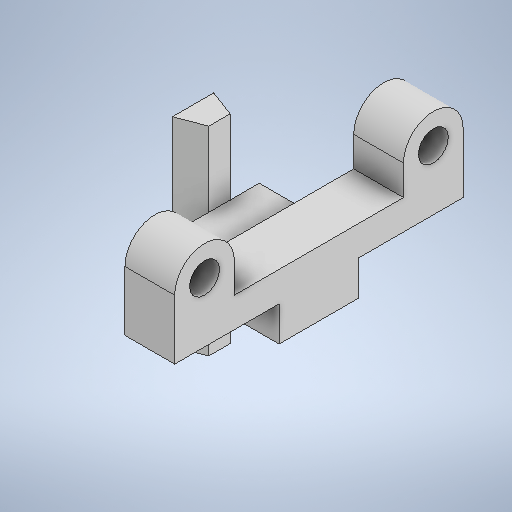
# Autodesk Inventor part: pelvis øvre del
Saved by Autodesk Inventor 2025.1 (Build 291241020, 241B)
## iProperties
Created: 2024-10-22
Part Number: pelvis øvre del
Material: Generic
Document SubType Name: Modeling
Designer: morte
Density: 1 g/cm^3
Appearance: Default
Author: morte
Autodesk Inventor part; units mm, degrees
ref_plane "YZ Plane" through (0, 0, 0) normal (1, 0, 0) x (0, 1, 0)
ref_plane "XZ Plane" through (0, 0, 0) normal (0, 1, 0) x (-1, 0, 0)
ref_plane "XY Plane" through (0, 0, 0) normal (0, 0, 1) x (1, 0, 0)
sketch "Sketch1" plane through (0, 0, 0) normal (1, 0, 0) x (0, 1, 0)
  line L0 (0, 0) -> (0, 8.5)
  line L1 (0, 14.5) -> (6, 14.5)
  line L2 (0, 0) -> (0, -8.5)
  line L3 (0, -14.5) -> (6, -14.5)
  line L4 (6, -14.5) -> (6, -8.5)
  line L5 (6, -8.5) -> (0, -8.5)
  line L6 (6, 14.5) -> (6, 8.5)
  line L7 (6, 8.5) -> (0, 8.5)
  line L8 (0, 14.5) -> (-3, 14.5)
  line L9 (-3, 14.5) -> (-3, -14.5)
  line L10 (-3, -14.5) -> (0, -14.5)
  line L11 (0, -8.5) -> (-3, -8.5)
  line L12 (0, 8.5) -> (-3, 8.5)
  line L13 (-3, 0) -> (-3, -5)
  dimension "d0" = 14.5
  dimension "d1" = 6
  dimension "d2" = 14.5
  dimension "d3" = 6
  dimension "d4" = 90
  dimension "d5" = 29
  dimension "d6" = 6
  dimension "d7" = 6
  dimension "d8" = 3
  dimension "d9" = 5
  constraints: 28 end point, 7 perpendicular, 4 point on line, 3 vertical, 1 collinear, 1 horizontal, 1 midpoint
  measures "d0" distance of L0.start L1.start
  measures "d1" distance of L1.start L1.end
  measures "d2" distance of L0.start L3.start
  measures "d3" distance of L3.start L3.end
  measures "d4" angle of L3 L2
  measures "d5" distance of L3.start L1.start
  measures "d6" distance of L3.end L4.end
  measures "d7" distance of L1.end L6.end
  measures "d8" distance of L1.start L8.end
  measures "d9" distance of L13.start L13.end
extrude "Extrusion1" add sketch "Sketch1" along normal mid plane 5
sketch "Sketch2" plane through (2.5, 0, 0) normal (1, 0, 0) x (0, 0, -1)
  line L0 (8.5, 0) -> (-8.5, 0) projected
  line L1 (0, 0) -> (-8.5, 0)
  line L2 (-8.5, 0) -> (-11.5, 0)
  line L3 (-14.5, 6) -> (-14.5, -3) projected
  line L4 (-11.5, 0) -> (-11.5, 3)
  line L5 (8.5, 0) -> (11.5, 0)
  line L6 (11.5, 0) -> (11.5, 3)
  circle A0 centre (-11.5, 3) radius 1.5
  circle A1 centre (11.5, 3) radius 1.5
  dimension "d14" = 3
  dimension "d15" = 3
  dimension "d16" = 3
  dimension "d17" = 3
  dimension "d18" = 3
  dimension "d19" = 3
  constraints: 10 end point, 3 perpendicular, 2 centre point, 2 coincident, 1 collinear, 1 horizontal
  measures "d14" distance of L0.end L2.end
  measures "d15" distance of L2.end L4.end
  measures "d16" distance of L0.start L5.end
  measures "d17" distance of L5.end L6.end
  measures "d18" diameter of A0
  measures "d19" diameter of A1
extrude "Extrusion2" cut sketch "Sketch2" against normal blind 10
sketch "Sketch3" plane through (-2.5, 0, 0) normal (-1, 0, 0) x (0, 0, 1)
  circle A0 centre (-11.5, 3) radius 1.5 projected
  circle A1 centre (-11.5, 3) radius 3
  line L0 (-14.5, 3) -> (-14.5, 7.7039)
  line L1 (-14.5, -3) -> (-14.5, 6) projected
  line L2 (-14.5, 7.7039) -> (-8.5, 7.7039)
  line L3 (-8.5, 7.7039) -> (-8.5, 3)
  circle A2 centre (11.5, 3) radius 1.5 projected
  circle A3 centre (11.5, 3) radius 3
  line L4 (8.5, 3) -> (8.5, 6.9796)
  line L5 (8.5, 6.9796) -> (14.5, 6.9796)
  line L6 (14.5, 6.9796) -> (14.5, 3)
  line L7 (14.5, 6) -> (14.5, -3) projected
  point P0 (0, 0)
  constraints: 12 end point, 4 point on circle, 2 centre point, 2 coincident, 2 perpendicular, 2 tangent, 1 collinear, 1 point on line, 1 vertical
extrude "Extrusion3" cut sketch "Sketch3" against normal through all contours A1 L0 L2 L3 | A3 L4 L5 L6
sketch "Sketch4" plane through (2.5, 0, 0) normal (1, 0, 0) x (0, 0, -1)
  line L0 (14.5, -3) -> (-14.5, -3) projected
  line L1 (0, -3) -> (4, -3)
  line L2 (0, -3) -> (-4, -3)
  line L3 (-4, -3) -> (-4, -1.5)
  line L4 (-4, -1.5) -> (4, -1.5)
  line L5 (4, -1.5) -> (4, -6.5)
  line L6 (4, -6.5) -> (-4, -6.5)
  line L7 (-4, -6.5) -> (-4, -1.5)
  point P0 (0, 0)
  dimension "d24" = 4
  dimension "d25" = 4
  dimension "d26" = 1.5
  dimension "d27" = 5
  dimension "d28" = 8
  constraints: 14 end point, 3 perpendicular, 3 point on line, 1 collinear, 1 midpoint
  measures "d24" distance of L1.start L1.end
  measures "d25" distance of L1.start L2.end
  measures "d26" distance of L2.end L3.end
  measures "d27" distance of L4.end L5.end
  measures "d28" distance of L5.end L6.end
extrude "Extrusion4" add sketch "Sketch4" against normal blind 10
sketch "Sketch24" plane through (-7.5, -1.5, -4) normal (0, 1, 0) x (1, 0, 0)
  line L0 (0, -8) -> (0, 0) projected
  line L1 (0, 0) -> (0, -4)
  line L2 (5, -8) -> (0, -8) projected
  line L3 (0, -4) -> (0, -5.075)
  line L4 (0, -4) -> (0, -2.925)
  line L5 (0, -4) -> (-2.65, -4)
  line L6 (-2.65, -4) -> (-2.65, -6.075)
  line L7 (-2.65, -4) -> (-0.575, -4) construction
  line L8 (-2.65, -4) -> (-2.65, -1.925)
  line L9 (-2.65, -1.925) -> (0, -2.925)
  line L10 (0, -5.075) -> (-2.65, -6.075)
  point P0 (7.5, -4)
  dimension "d150" = 4
  dimension "d151" = 1.075
  dimension "d152" = 1.075
  dimension "d153" = 2.65
  dimension "d154" = 2.075
  dimension "d155" = 90
  dimension "d156" = 2.075
  constraints: 18 end point, 3 perpendicular, 2 point on line, 2 vertical, 1 horizontal
  measures "d150" distance of L0.end L1.end
  measures "d151" distance of L1.end L3.end
  measures "d152" distance of L1.end L4.end
  measures "d153" distance of L1.end L5.end
  measures "d154" distance of L5.end L6.end
  measures "d155" angle of L6 L7
  measures "d156" distance of L5.end L8.end
extrude "Extrusion20" add sketch "Sketch24" along normal mid plane 15
sketch "Sketch25" plane through (2.5, -6.5, -4) normal (0, -1, 0) x (1, 0, 0)
  line L0 (-10, 2.925) -> (-12.65, 1.925) projected
  line L1 (-12.65, 1.925) -> (-12.65, 6.075) projected
  line L2 (-12.65, 1.925) -> (-12.65, 6.075)
  line L3 (-10, 8) -> (-10, 5.075) projected
  line L4 (-12.65, 6.075) -> (-10, 5.075)
  line L5 (-10, 5.075) -> (-10, 2.925) projected
  line L6 (-10, 5.075) -> (-10, 2.925)
  line L7 (-10, 2.925) -> (-12.65, 1.925)
  point P0 (-2.5, 4)
  constraints: 8 end point, 1 collinear, 1 vertical
extrude "Extrusion21" add sketch "Sketch25" along normal blind 7.5
body "Solid1"
